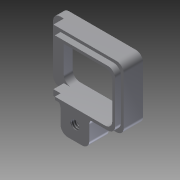
# Autodesk Inventor part: window_f
Saved by Autodesk Inventor 2011 (Build 150239000, 239)
## iProperties
Created: 2011-05-24
Part Number: window_f
Document SubType Name: Modeling
Designer: labuser
Density: 1 g/cm^3
Author: labuser
Autodesk Inventor part; units mm, degrees
ref_plane "YZ Plane" through (0, 0, 0) normal (1, 0, 0) x (0, 1, 0)
ref_plane "XZ Plane" through (0, 0, 0) normal (0, 1, 0) x (-1, 0, 0)
ref_plane "XY Plane" through (0, 0, 0) normal (0, 0, 1) x (1, 0, 0)
sketch "Sketch1" plane through (0, 0, 0) normal (0, 0, 1) x (1, 0, 0)
  circle A0 centre (0, 0) radius 3.5 construction
  circle A1 centre (0, 0) radius 4.5 construction
  line L0 (0, 0) -> (4.5, 0) construction
  line L1 (4.5, 0) -> (4.5, 3.5) construction
  line L2 (4.5, 3.5) -> (0, 3.5) construction
  line L3 (0, 3.5) -> (0, 0) construction
  line L4 (4.5, 3.5) -> (-4.5, 3.5)
  line L5 (-4.5, 3.5) -> (-4.5, -3.5)
  line L6 (-4.5, -3.5) -> (4.5, -3.5)
  line L7 (4.5, -3.5) -> (4.5, 3.5)
  line L8 (-4.5, 3.5) -> (-6, 3.5) construction
  line L9 (-6, 3.5) -> (-6, -3.5) construction
  line L10 (-6, -3.5) -> (-4.5, -3.5) construction
  line L11 (-4.5, -3.5) -> (-4.5, 3.5) construction
  line L12 (-6, 3.5) -> (4.5, 3.5) construction
  line L13 (4.5, 3.5) -> (4.5, 4.3) construction
  line L14 (4.5, 4.3) -> (-6, 4.3) construction
  line L15 (-6, 4.3) -> (-6, 3.5) construction
  line L16 (-6, -3.5) -> (4.5, -3.5) construction
  line L17 (4.5, -3.5) -> (4.5, -4.3) construction
  line L18 (4.5, -4.3) -> (-6, -4.3) construction
  line L19 (-6, -4.3) -> (-6, -3.5) construction
  line L20 (4.5, -4.3) -> (5.3, -4.3) construction
  line L21 (5.3, -4.3) -> (5.3, 4.3) construction
  line L22 (5.3, 4.3) -> (4.5, 4.3) construction
  line L23 (4.5, 4.3) -> (4.5, -4.3) construction
  line L24 (-6, 4.3) -> (5.3, 4.3)
  line L25 (5.3, 4.3) -> (5.3, -4.3)
  line L26 (5.3, -4.3) -> (-6, -4.3)
  line L27 (-6, -4.3) -> (-6, 4.3)
  dimension "d0" = 7
  dimension "d1" = 9
  dimension "d2" = 4.5
  dimension "d3" = 3.5
  dimension "d4" = 1.5
  dimension "d5" = 0.8
  dimension "d6" = 0.8
  dimension "d7" = 0.8
  constraints: 56 end point, 14 parallel, 7 horizontal, 7 perpendicular, 2 centre point, 2 coincident
  measures "d0" diameter of A0
  measures "d1" diameter of A1
  measures "d2" distance of L2.end L1.end
  measures "d3" distance of L1.end L0.end
  measures "d4" distance of L10.end L9.end
  measures "d5" distance of L13.end L12.end
  measures "d6" distance of L16.end L17.end
  measures "d7" distance of L22.end L21.end
extrude "Extrusion1" add sketch "Sketch1" along normal blind 3.5
sketch "Sketch2" plane through (0, 0, 3.5) normal (0, 0, 1) x (1, 0, 0)
  line L0 (5.3, -4.3) -> (-6, -4.3) projected
  line L1 (-6, 4.3) -> (-4.5, 4.3)
  line L2 (-4.5, 4.3) -> (-4.5, -4.3)
  line L3 (-4.5, -4.3) -> (-6, -4.3)
  line L4 (-6, -4.3) -> (-6, 4.3)
  point P0 (0, 0)
  constraints: 8 end point, 2 parallel, 1 horizontal, 1 perpendicular, 1 point on line
extrude "Extrusion2" cut sketch "Sketch2" against normal blind 2.25
sketch "Sketch3" plane through (0, 0, 3.5) normal (0, 0, 1) x (1, 0, 0)
  line L0 (-4.5, -3.5) -> (-4.5, -4.3) projected
  line L1 (5.3, -4.3) -> (-4.5, -4.3) projected
  line L2 (5.3, 4.3) -> (5.3, -4.3) projected
  line L3 (-4.5, 4.3) -> (5.3, 4.3) construction
  line L4 (5.3, 4.3) -> (5.3, 3.9) construction
  line L5 (5.3, 3.9) -> (-4.5, 3.9) construction
  line L6 (-4.5, 3.9) -> (-4.5, 4.3) construction
  line L7 (5.3, 4.3) -> (4.9, 4.3) construction
  line L8 (4.9, 4.3) -> (4.9, -4.3) construction
  line L9 (4.9, -4.3) -> (5.3, -4.3) construction
  line L10 (5.3, -4.3) -> (5.3, 4.3) construction
  line L11 (5.3, -4.3) -> (-4.5, -4.3) construction
  line L12 (-4.5, -4.3) -> (-4.5, -3.9) construction
  line L13 (-4.5, -3.9) -> (5.3, -3.9) construction
  line L14 (5.3, -3.9) -> (5.3, -4.3) construction
  line L15 (-4.5, 3.9) -> (-4.5, 4.3)
  line L16 (5.3, 4.3) -> (5.3, -4.3)
  line L17 (-4.5, -4.3) -> (-4.5, -3.9)
  line L18 (4.9, -3.9) -> (4.9, 3.9)
  line L19 (4.9, 3.9) -> (-4.5, 3.9)
  line L20 (-4.5, 4.3) -> (5.3, 4.3)
  line L21 (4.9, -3.9) -> (-4.5, -3.9)
  line L22 (-4.5, -4.3) -> (5.3, -4.3)
  point P0 (0, 0)
  dimension "d12" = 0.4
  dimension "d13" = 0.4
  dimension "d14" = 0.4
  constraints: 40 end point, 11 parallel, 6 point on line, 3 horizontal, 3 perpendicular, 2 collinear, 1 midpoint
  measures "d12" distance of L3.end L4.end
  measures "d13" distance of L9.end L8.end
  measures "d14" distance of L11.end L12.end
extrude "Extrusion3" cut sketch "Sketch3" against normal blind 0.8
sketch "Sketch4" plane through (-6, -4.3, 0) normal (0, -1, 0) x (1, 0, 0)
  line L0 (11.3, 2.7) -> (1.5, 2.7) projected
  line L1 (11.3, 0) -> (0, 0) projected
  line L2 (12.285, 1.4959) -> (-1.3636, 1.4959) construction
  line L3 (6, 1.4959) -> (8, 1.4959) construction
  line L4 (8, 2.7) -> (6, 2.7) construction
  line L5 (8, 2.7) -> (4, 2.7)
  line L6 (1.5, 2.7) -> (2.5, 2.7) construction
  line L7 (2.5, 2.7) -> (2.5, 0) construction
  line L8 (2.5, 0) -> (1.5, 0) construction
  line L9 (1.5, 0) -> (1.5, 2.7) construction
  line L10 (2.5, 2.7) -> (6.5, 2.7)
  line L11 (6.5, 2.7) -> (6.5, 0)
  line L12 (6.5, 0) -> (2.5, 0)
  line L13 (2.5, 0) -> (2.5, 2.7)
  point P0 (6, 0)
  point P1 (4, 0)
  dimension "d29" = 1
  dimension "d30" = 4
  constraints: 24 end point, 5 parallel, 5 point on line, 4 horizontal, 2 perpendicular
  measures "d29" distance of L7.end L8.end
  measures "d30" distance of L11.end L12.end
extrude "Extrusion4" add sketch "Sketch4" along normal blind 4
fillet "Fillet1" radius 1 14 edges at (5.3, -4.3, 1.35) (4.9, -3.9, 3.1) (-6, -4.3, 0.625) (-6, 4.3, 0.625) (4.9, 3.9, 3.1) (5.3, 4.3, 1.35) (-3.5, -4.3, 1.35) (0.5, -4.3, 1.35) (0.5, -8.3, 1.35) (-3.5, -8.3, 1.35) (4.5, 3.5, 1.75) (4.5, -3.5, 1.75) (-4.5, 3.5, 0.625) (-4.5, -3.5, 0.625)
sketch "Sketch6" plane through (0, 0, 2.7) normal (0, 0, 1) x (1, 0, 0)
  point P0 (0, 0)
  point P1 (-1.5, -6.3)
hole "Hole2" at (-1.5, -6.3, 2.7) direction (0, 0, -1) diameter 1.1938 end through all
sketch "Sketch7" plane through (-4.5, 3.5, 1.25) normal (-1, 0, 0) x (0, 0, 1)
  line L0 (0, 0) -> (2.25, 0) projected
  line L1 (2.25, 0.4) -> (1.45, 0.4)
  line L2 (1.45, 0.4) -> (1.45, 0)
  line L3 (1.45, 0) -> (2.25, 0)
  line L4 (2.25, 0) -> (2.25, 0.4)
  point P0 (-1.25, -3.5)
  constraints: 8 end point, 2 parallel, 1 horizontal, 1 perpendicular, 1 point on line
extrude "Extrusion5" cut sketch "Sketch7" against normal blind 1
sketch "Sketch8" plane through (-4.5, -3.5, 1.25) normal (-1, 0, 0) x (0, 0, 1)
  line L0 (2.25, 0) -> (1.45, 0)
  line L1 (1.45, 0) -> (1.45, -0.4)
  line L2 (1.45, -0.4) -> (2.25, -0.4)
  line L3 (2.25, -0.4) -> (2.25, 0)
  point P0 (-1.25, 3.5)
  constraints: 8 end point, 2 parallel, 1 horizontal, 1 perpendicular
extrude "Extrusion6" cut sketch "Sketch8" against normal blind 1
body "Solid1"
